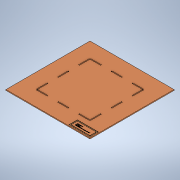
# Autodesk Inventor part: BasePlate_V1
Saved by Autodesk Inventor 2022.2 (Build 262287000, 287)
## iProperties
Created: 2022-11-15
Part Number: BasePlate_V1
Material: Generic
Document SubType Name: Modeling
Designer: jaege
Density: 1 g/cm^3
Appearance: Red Oak - Natural Low Gloss
Author: jaege
Autodesk Inventor part; units mm, degrees
(part 1 of 2)
ref_plane "YZ Plane" through (0, 0, 0) normal (1, 0, 0) x (0, 1, 0)
ref_plane "XZ Plane" through (0, 0, 0) normal (0, 1, 0) x (-1, 0, 0)
ref_plane "XY Plane" through (0, 0, 0) normal (0, 0, 1) x (1, 0, 0)
sketch "Sketch1" plane through (0, 0, 0) normal (0, 1, 0) x (-1, 0, 0)
  line L0 (200, -200) -> (-200, -200)
  line L1 (-200, -200) -> (-200, 200)
  line L2 (-200, 200) -> (200, 200)
  line L3 (200, 200) -> (200, -200)
  line L4 (200, -200) -> (-200, 200) construction
  line L5 (-200, -200) -> (200, 200) construction
  line L6 (-125, -125) -> (125, -125) construction
  line L7 (125, -125) -> (125, 125) construction
  line L8 (125, 125) -> (-125, 125) construction
  line L9 (-125, 125) -> (-125, -125) construction
  line L10 (-125, -125) -> (125, 125) construction
  line L11 (125, -125) -> (-125, 125) construction
  line L12 (125, 125) -> (129, 125)
  line L13 (129, 125) -> (129, 75)
  line L14 (129, 75) -> (125, 75)
  line L15 (125, 75) -> (125, 125)
  line L16 (125, 75) -> (129, 75)
  line L17 (125, 25) -> (125, 75) construction
  line L18 (129, 75) -> (129, 25) construction
  line L19 (129, 25) -> (125, 25)
  line L20 (125, 25) -> (129, 25)
  line L21 (125, -25) -> (125, 25)
  line L22 (129, 25) -> (129, -25)
  line L23 (129, -25) -> (125, -25)
  line L24 (125, -25) -> (129, -25)
  line L25 (125, -75) -> (125, -25) construction
  line L26 (129, -25) -> (129, -75) construction
  line L27 (129, -75) -> (125, -75)
  line L28 (125, -75) -> (129, -75)
  line L29 (125, -125) -> (125, -75)
  line L30 (129, -75) -> (129, -125)
  line L31 (129, -125) -> (125, -125)
  line L32 (125, 125) -> (75, 125)
  line L33 (75, 125) -> (75, 129)
  line L34 (75, 129) -> (125, 129)
  line L35 (125, 129) -> (125, 125)
  line L36 (125, -125) -> (75, -125)
  line L37 (75, -125) -> (75, -129)
  line L38 (75, -129) -> (125, -129)
  line L39 (125, -129) -> (125, -125)
  line L40 (75, 125) -> (25, 125) construction
  line L41 (75, 129) -> (75, 125)
  line L42 (25, 129) -> (75, 129) construction
  line L43 (25, 125) -> (25, 129)
  line L44 (75, -125) -> (25, -125) construction
  line L45 (25, -125) -> (25, -129)
  line L46 (25, -129) -> (75, -129) construction
  line L47 (75, -129) -> (75, -125)
  line L48 (25, 125) -> (-25, 125)
  line L49 (25, 129) -> (25, 125)
  line L50 (-25, 129) -> (25, 129)
  line L51 (-25, 125) -> (-25, 129)
  line L52 (25, -125) -> (-25, -125)
  line L53 (-25, -125) -> (-25, -129)
  line L54 (-25, -129) -> (25, -129)
  line L55 (25, -129) -> (25, -125)
  line L56 (-25, 125) -> (-75, 125) construction
  line L57 (-25, 129) -> (-25, 125)
  line L58 (-75, 129) -> (-25, 129) construction
  line L59 (-75, 125) -> (-75, 129)
  line L60 (-25, -125) -> (-75, -125) construction
  line L61 (-75, -125) -> (-75, -129)
  line L62 (-75, -129) -> (-25, -129) construction
  line L63 (-25, -129) -> (-25, -125)
  line L64 (-75, 125) -> (-125, 125)
  line L65 (-75, 129) -> (-75, 125)
  line L66 (-125, 129) -> (-75, 129)
  line L67 (-125, 125) -> (-125, 129)
  line L68 (-75, -125) -> (-125, -125)
  line L69 (-125, -125) -> (-125, -129)
  line L70 (-125, -129) -> (-75, -129)
  line L71 (-75, -129) -> (-75, -125)
  line L72 (-125, 125) -> (-129, 125)
  line L73 (-129, 125) -> (-129, 75)
  line L74 (-129, 75) -> (-125, 75)
  line L75 (-125, 75) -> (-125, 125)
  line L76 (-125, 25) -> (-125, 75)
  line L77 (-129, 25) -> (-125, 25)
  line L78 (-129, 75) -> (-129, 25) construction
  line L79 (-125, 75) -> (-129, 75)
  line L80 (-125, -25) -> (-125, 25)
  line L81 (-129, -25) -> (-125, -25)
  line L82 (-129, 25) -> (-129, -25)
  line L83 (-125, 25) -> (-129, 25)
  line L84 (-125, -75) -> (-125, -25) construction
  line L85 (-129, -75) -> (-125, -75)
  line L86 (-129, -25) -> (-129, -75) construction
  line L87 (-125, -25) -> (-129, -25)
  line L88 (-125, -125) -> (-125, -75)
  line L89 (-129, -125) -> (-125, -125)
  line L90 (-129, -75) -> (-129, -125)
  line L91 (-125, -75) -> (-129, -75)
  point P0 (0, 0)
  point P1 (75, -125)
  point P2 (25, -125)
  point P3 (-25, -125)
  point P4 (-75, -125)
  dimension "d0" = 400
  dimension "d1" = 400
  dimension "d2" = 250
  dimension "d3" = 250
  dimension "d4" = 4
  dimension "d5" = 50
  dimension "d8" = 50
  dimension "d13" = 50
  dimension "d14" = 4
  dimension "d15" = 50
  dimension "d16" = 4
  dimension "d19" = 50
  dimension "d24" = 4
  dimension "d25" = 50
  dimension "d28" = 50
  constraints: 184 end point, 12 parallel, 7 horizontal, 6 perpendicular, 4 midpoint, 2 vertical, 136 other
  measures "d0" distance of L1.end L2.end
  measures "d1" distance of L0.end L1.end
  measures "d2" distance of L8.end L7.end
  measures "d3" distance of L7.end L6.end
  measures "d4" distance of L13.end L14.end
  measures "d5" distance of L12.end L13.end
  measures "d8" distance of L12.end L16.end
  measures "d13" distance of L33.end L34.end
  measures "d14" distance of L32.end L33.end
  measures "d15" distance of L38.end L37.end
  measures "d16" distance of L37.end L36.end
  measures "d19" distance of L7.end L40.start
  measures "d24" distance of L74.end L73.end
  measures "d25" distance of L73.end L72.end
  measures "d28" distance of L74.end L76.start
extrude "Extrusion1" add sketch "Sketch1" along normal blind 4
sketch "Sketch2" plane through (0, 4, 0) normal (0, 1, 0) x (1, 0, 0)
  line L0 (-200, -200) -> (200, -200) projected
  line L1 (200, -200) -> (90, -200) construction
  line L2 (90, -200) -> (90, -150) construction
  line L3 (90, -150) -> (200, -150) construction
  line L4 (200, -150) -> (200, -200) construction
  line L5 (195, -155) -> (95, -155)
  line L6 (95, -155) -> (95, -195)
  line L7 (95, -195) -> (195, -195)
  line L8 (195, -195) -> (195, -155)
  line L9 (100, -160) -> (190, -160)
  line L10 (190, -160) -> (190, -190)
  line L11 (190, -190) -> (100, -190)
  line L12 (100, -190) -> (100, -160)
  line L13 (110, -168.25) -> (180, -168.25) construction
  line L14 (180, -168.25) -> (180, -181.75) construction
  line L15 (180, -181.75) -> (110, -181.75) construction
  line L16 (110, -181.75) -> (110, -168.25) construction
  line L17 (110, -168.25) -> (180, -181.75) construction
  line L18 (100, -190) -> (190, -160) construction
  spline S0 degree 2 poles (112.3777, -170.519) (112.3777, -170.7464) (112.2047, -171.0949) (112.0613, -171.2085) knots 0 0 0 1 2 2 2
  spline S1 degree 2 poles (112.0613, -171.2085) (111.8883, -171.342) (111.4953, -171.4557) (111.1839, -171.4557) knots 0 0 0 1 2 2 2
  line L19 (111.1839, -171.4557) -> (110.309, -171.4557)
  line L20 (110.309, -171.4557) -> (110.309, -168.4057)
  line L21 (110.309, -168.4057) -> (111.1172, -168.4057)
  spline S2 degree 2 poles (111.1172, -168.4057) (111.4434, -168.4057) (111.7697, -168.4477) (111.918, -168.5293) knots 0 0 0 1 2 2 2
  spline S3 degree 2 poles (111.918, -168.5293) (112.0836, -168.6158) (112.2344, -168.9) (112.2344, -169.0928) knots 0 0 0 1 2 2 2
  spline S4 degree 2 poles (112.2344, -169.0928) (112.2344, -169.3079) (112.007, -169.6489) (111.8068, -169.7453) knots 0 0 0 1 2 2 2
  line L22 (111.8068, -169.7453) -> (111.8068, -169.7602)
  spline S5 degree 2 poles (111.8068, -169.7602) (112.0786, -169.8343) (112.3777, -170.2273) (112.3777, -170.519) knots 0 0 0 1 2 2 2
  spline S6 degree 2 poles (111.9551, -170.5363) (111.9551, -170.3632) (111.8562, -170.1408) (111.7079, -170.0617) knots 0 0 0 1 2 2 2
  spline S7 degree 2 poles (111.7079, -170.0617) (111.6115, -170.0123) (111.3841, -169.9826) (111.174, -169.9826) knots 0 0 0 1 2 2 2
  line L23 (111.174, -169.9826) -> (110.7143, -169.9826)
  line L24 (110.7143, -169.9826) -> (110.7143, -171.1097)
  line L25 (110.7143, -171.1097) -> (111.043, -171.1097)
  spline S8 degree 2 poles (111.043, -171.1097) (111.31, -171.1097) (111.6165, -171.0603) (111.7351, -170.9812) knots 0 0 0 1 2 2 2
  spline S9 degree 2 poles (111.7351, -170.9812) (111.8488, -170.8996) (111.9551, -170.6969) (111.9551, -170.5363) knots 0 0 0 1 2 2 2
  spline S10 degree 2 poles (111.8117, -169.1497) (111.8117, -169.0409) (111.7376, -168.8778) (111.656, -168.8308) knots 0 0 0 1 2 2 2
  spline S11 degree 2 poles (111.656, -168.8308) (111.5571, -168.7765) (111.3174, -168.7517) (111.1024, -168.7517) knots 0 0 0 1 2 2 2
  line L26 (111.1024, -168.7517) -> (110.7143, -168.7517)
  line L27 (110.7143, -168.7517) -> (110.7143, -169.644)
  line L28 (110.7143, -169.644) -> (111.174, -169.644)
  spline S12 degree 2 poles (111.174, -169.644) (111.3643, -169.644) (111.5448, -169.6045) (111.6412, -169.5427) knots 0 0 0 1 2 2 2
  spline S13 degree 2 poles (111.6412, -169.5427) (111.7351, -169.4833) (111.8117, -169.293) (111.8117, -169.1497) knots 0 0 0 1 2 2 2
  spline S14 degree 2 poles (114.0263, -171.2135) (113.9793, -171.2481) (113.8212, -171.3717) (113.747, -171.4088) knots 0 0 0 1 2 2 2
  spline S15 degree 2 poles (113.747, -171.4088) (113.6457, -171.4631) (113.4553, -171.52) (113.2823, -171.52) knots 0 0 0 1 2 2 2
  spline S16 degree 2 poles (113.2823, -171.52) (113.1415, -171.52) (112.8869, -171.4137) (112.7905, -171.3173) knots 0 0 0 1 2 2 2
  spline S17 degree 2 poles (112.7905, -171.3173) (112.699, -171.2234) (112.5878, -170.9466) (112.5878, -170.7933) knots 0 0 0 1 2 2 2
  spline S18 degree 2 poles (112.5878, -170.7933) (112.5878, -170.556) (112.788, -170.2199) (113.0055, -170.1235) knots 0 0 0 1 2 2 2
  spline S19 degree 2 poles (113.0055, -170.1235) (113.1983, -170.0345) (113.7223, -169.9678) (114.0263, -169.9505) knots 0 0 0 1 2 2 2
  line L29 (114.0263, -169.9505) -> (114.0263, -169.8763)
  spline S20 degree 2 poles (114.0263, -169.8763) (114.0263, -169.7429) (113.9447, -169.5773) (113.8706, -169.5303) knots 0 0 0 1 2 2 2
  spline S21 degree 2 poles (113.8706, -169.5303) (113.7964, -169.4833) (113.5839, -169.4537) (113.4702, -169.4537) knots 0 0 0 1 2 2 2
  spline S22 degree 2 poles (113.4702, -169.4537) (113.3367, -169.4537) (112.9759, -169.5328) (112.7954, -169.6094) knots 0 0 0 1 2 2 2
  line L30 (112.7954, -169.6094) -> (112.7732, -169.6094)
  line L31 (112.7732, -169.6094) -> (112.7732, -169.2164)
  spline S23 degree 2 poles (112.7732, -169.2164) (112.8795, -169.1868) (113.2774, -169.1126) (113.4727, -169.1126) knots 0 0 0 1 2 2 2
  spline S24 degree 2 poles (113.4727, -169.1126) (113.7099, -169.1126) (114.0337, -169.1868) (114.1622, -169.2831) knots 0 0 0 1 2 2 2
  spline S25 degree 2 poles (114.1622, -169.2831) (114.2883, -169.3771) (114.4119, -169.6761) (114.4119, -169.8912) knots 0 0 0 1 2 2 2
  line L32 (114.4119, -169.8912) -> (114.4119, -171.4557)
  line L33 (114.4119, -171.4557) -> (114.0263, -171.4557)
  line L34 (114.0263, -171.4557) -> (114.0263, -171.2135)
  line L35 (114.0263, -170.8922) -> (114.0263, -170.257)
  spline S26 degree 2 poles (114.0263, -170.257) (113.8879, -170.2693) (113.4702, -170.3113) (113.3392, -170.3509) knots 0 0 0 1 2 2 2
  spline S27 degree 2 poles (113.3392, -170.3509) (113.1859, -170.3979) (112.9857, -170.5931) (112.9857, -170.7661) knots 0 0 0 1 2 2 2
  spline S28 degree 2 poles (112.9857, -170.7661) (112.9857, -170.9639) (113.2082, -171.1641) (113.4207, -171.1641) knots 0 0 0 1 2 2 2
  spline S29 degree 2 poles (113.4207, -171.1641) (113.6012, -171.1641) (113.8978, -171.0083) (114.0263, -170.8922) knots 0 0 0 1 2 2 2
  spline S30 degree 2 poles (115.8627, -171.5076) (115.6254, -171.5076) (115.2325, -171.3618) (115.0916, -171.2135) knots 0 0 0 1 2 2 2
  spline S31 degree 2 poles (115.0916, -171.2135) (114.9507, -171.0677) (114.795, -170.6178) (114.795, -170.3163) knots 0 0 0 1 2 2 2
  spline S32 degree 2 poles (114.795, -170.3163) (114.795, -170.0147) (114.9556, -169.5748) (115.0916, -169.4265) knots 0 0 0 1 2 2 2
  spline S33 degree 2 poles (115.0916, -169.4265) (115.2275, -169.2757) (115.6304, -169.1151) (115.8627, -169.1151) knots 0 0 0 1 2 2 2
  spline S34 degree 2 poles (115.8627, -169.1151) (116.0506, -169.1151) (116.4015, -169.2214) (116.5375, -169.2906) knots 0 0 0 1 2 2 2
  line L36 (116.5375, -169.2906) -> (116.5375, -169.7231)
  line L37 (116.5375, -169.7231) -> (116.5152, -169.7231)
  spline S35 degree 2 poles (116.5152, -169.7231) (116.4732, -169.6885) (116.3447, -169.5995) (116.2532, -169.5526) knots 0 0 0 1 2 2 2
  spline S36 degree 2 poles (116.2532, -169.5526) (116.1717, -169.513) (115.9542, -169.4512) (115.8553, -169.4512) knots 0 0 0 1 2 2 2
  spline S37 degree 2 poles (115.8553, -169.4512) (115.5562, -169.4512) (115.1929, -169.9035) (115.1929, -170.3163) knots 0 0 0 1 2 2 2
  spline S38 degree 2 poles (115.1929, -170.3163) (115.1929, -170.7192) (115.5439, -171.1715) (115.8553, -171.1715) knots 0 0 0 1 2 2 2
  spline S39 degree 2 poles (115.8553, -171.1715) (116.0432, -171.1715) (116.3842, -171.0158) (116.5152, -170.8947) knots 0 0 0 1 2 2 2
  line L38 (116.5152, -170.8947) -> (116.5375, -170.8947)
  line L39 (116.5375, -170.8947) -> (116.5375, -171.3272)
  spline S40 degree 2 poles (116.5375, -171.3272) (116.4806, -171.3544) (116.3076, -171.431) (116.2384, -171.4483) knots 0 0 0 1 2 2 2
  spline S41 degree 2 poles (116.2384, -171.4483) (116.1395, -171.478) (115.9838, -171.5076) (115.8627, -171.5076) knots 0 0 0 1 2 2 2
  line L40 (118.6853, -171.4557) -> (118.2998, -171.4557)
  line L41 (118.2998, -171.4557) -> (118.2998, -170.1507)
  spline S42 degree 2 poles (118.2998, -170.1507) (118.2998, -169.9925) (118.2701, -169.7206) (118.2256, -169.6391) knots 0 0 0 1 2 2 2
  spline S43 degree 2 poles (118.2256, -169.6391) (118.1786, -169.5526) (118.0106, -169.4685) (117.8672, -169.4685) knots 0 0 0 1 2 2 2
  spline S44 degree 2 poles (117.8672, -169.4685) (117.7239, -169.4685) (117.4199, -169.6218) (117.274, -169.7453) knots 0 0 0 1 2 2 2
  line L42 (117.274, -169.7453) -> (117.274, -171.4557)
  line L43 (117.274, -171.4557) -> (116.8885, -171.4557)
  line L44 (116.8885, -171.4557) -> (116.8885, -168.2698)
  line L45 (116.8885, -168.2698) -> (117.274, -168.2698)
  line L46 (117.274, -168.2698) -> (117.274, -169.4216)
  spline S45 degree 2 poles (117.274, -169.4216) (117.447, -169.2658) (117.7807, -169.1027) (117.9686, -169.1027) knots 0 0 0 1 2 2 2
  spline S46 degree 2 poles (117.9686, -169.1027) (118.3047, -169.1027) (118.6853, -169.5476) (118.6853, -169.9703) knots 0 0 0 1 2 2 2
  line L47 (118.6853, -169.9703) -> (118.6853, -171.4557)
  spline S47 degree 2 poles (120.2202, -171.5076) (119.6715, -171.5076) (119.0684, -170.8922) (119.0684, -170.3237) knots 0 0 0 1 2 2 2
  spline S48 degree 2 poles (119.0684, -170.3237) (119.0684, -169.7651) (119.6542, -169.1027) (120.1263, -169.1027) knots 0 0 0 1 2 2 2
  spline S49 degree 2 poles (120.1263, -169.1027) (120.3389, -169.1027) (120.6676, -169.2263) (120.7887, -169.3573) knots 0 0 0 1 2 2 2
  spline S50 degree 2 poles (120.7887, -169.3573) (120.9123, -169.4883) (121.0433, -169.8665) (121.0433, -170.1408) knots 0 0 0 1 2 2 2
  line L48 (121.0433, -170.1408) -> (121.0433, -170.3509)
  line L49 (121.0433, -170.3509) -> (119.459, -170.3509)
  spline S51 degree 2 poles (119.459, -170.3509) (119.459, -170.7488) (119.8594, -171.1715) (120.2153, -171.1715) knots 0 0 0 1 2 2 2
  spline S52 degree 2 poles (120.2153, -171.1715) (120.3413, -171.1715) (120.586, -171.1146) (120.6849, -171.0701) knots 0 0 0 1 2 2 2
  spline S53 degree 2 poles (120.6849, -171.0701) (120.7887, -171.0207) (120.9321, -170.9342) (120.979, -170.8947) knots 0 0 0 1 2 2 2
  line L50 (120.979, -170.8947) -> (121.0013, -170.8947)
  line L51 (121.0013, -170.8947) -> (121.0013, -171.3148)
  spline S54 degree 2 poles (121.0013, -171.3148) (120.9345, -171.342) (120.7318, -171.4211) (120.6528, -171.4434) knots 0 0 0 1 2 2 2
  spline S55 degree 2 poles (120.6528, -171.4434) (120.5415, -171.4755) (120.3586, -171.5076) (120.2202, -171.5076) knots 0 0 0 1 2 2 2
  spline S56 degree 2 poles (120.6676, -170.0568) (120.6626, -169.9011) (120.5984, -169.6737) (120.5366, -169.597) knots 0 0 0 1 2 2 2
  spline S57 degree 2 poles (120.5366, -169.597) (120.4699, -169.5105) (120.2598, -169.4191) (120.1041, -169.4191) knots 0 0 0 1 2 2 2
  spline S58 degree 2 poles (120.1041, -169.4191) (119.9508, -169.4191) (119.7358, -169.5105) (119.6468, -169.5995) knots 0 0 0 1 2 2 2
  spline S59 degree 2 poles (119.6468, -169.5995) (119.5603, -169.691) (119.4713, -169.9109) (119.459, -170.0568) knots 0 0 0 1 2 2 2
  line L52 (119.459, -170.0568) -> (120.6676, -170.0568)
  line L53 (121.8268, -171.4557) -> (121.4412, -171.4557)
  line L54 (121.4412, -171.4557) -> (121.4412, -168.2698)
  line L55 (121.4412, -168.2698) -> (121.8268, -168.2698)
  line L56 (121.8268, -168.2698) -> (121.8268, -171.4557)
  spline S60 degree 2 poles (124.2737, -170.3113) (124.2737, -170.8897) (123.7176, -171.52) (123.2529, -171.52) knots 0 0 0 1 2 2 2
  spline S61 degree 2 poles (123.2529, -171.52) (122.7759, -171.52) (122.2297, -170.8699) (122.2297, -170.3113) knots 0 0 0 1 2 2 2
  spline S62 degree 2 poles (122.2297, -170.3113) (122.2297, -169.7379) (122.7932, -169.1027) (123.2529, -169.1027) knots 0 0 0 1 2 2 2
  spline S63 degree 2 poles (123.2529, -169.1027) (123.7176, -169.1027) (124.2737, -169.7355) (124.2737, -170.3113) knots 0 0 0 1 2 2 2
  spline S64 degree 2 poles (123.8758, -170.3113) (123.8758, -169.8665) (123.552, -169.4339) (123.2529, -169.4339) knots 0 0 0 1 2 2 2
  spline S65 degree 2 poles (123.2529, -169.4339) (122.9538, -169.4339) (122.6276, -169.8665) (122.6276, -170.3113) knots 0 0 0 1 2 2 2
  spline S66 degree 2 poles (122.6276, -170.3113) (122.6276, -170.7439) (122.9538, -171.1888) (123.2529, -171.1888) knots 0 0 0 1 2 2 2
  spline S67 degree 2 poles (123.2529, -171.1888) (123.5495, -171.1888) (123.8758, -170.7513) (123.8758, -170.3113) knots 0 0 0 1 2 2 2
  line L57 (125.8827, -169.5797) -> (125.863, -169.5797)
  spline S68 degree 2 poles (125.863, -169.5797) (125.8185, -169.5674) (125.7221, -169.5624) (125.6553, -169.5624) knots 0 0 0 1 2 2 2
  spline S69 degree 2 poles (125.6553, -169.5624) (125.4996, -169.5624) (125.1932, -169.6984) (125.0547, -169.8318) knots 0 0 0 1 2 2 2
  line L58 (125.0547, -169.8318) -> (125.0547, -171.4557)
  line L59 (125.0547, -171.4557) -> (124.6692, -171.4557)
  line L60 (124.6692, -171.4557) -> (124.6692, -169.167)
  line L61 (124.6692, -169.167) -> (125.0547, -169.167)
  line L62 (125.0547, -169.167) -> (125.0547, -169.5081)
  spline S70 degree 2 poles (125.0547, -169.5081) (125.2648, -169.3202) (125.5787, -169.167) (125.727, -169.167) knots 0 0 0 1 2 2 2
  spline S71 degree 2 poles (125.727, -169.167) (125.7863, -169.167) (125.8457, -169.1719) (125.8827, -169.1793) knots 0 0 0 1 2 2 2
  line L63 (125.8827, -169.1793) -> (125.8827, -169.5797)
  spline S72 degree 2 poles (128.0998, -170.2496) (128.0998, -170.823) (127.5536, -171.5002) (127.1359, -171.5002) knots 0 0 0 1 2 2 2
  spline S73 degree 2 poles (127.1359, -171.5002) (126.9653, -171.5002) (126.7033, -171.4211) (126.5674, -171.3395) knots 0 0 0 1 2 2 2
  line L64 (126.5674, -171.3395) -> (126.5674, -172.2985)
  line L65 (126.5674, -172.2985) -> (126.1818, -172.2985)
  line L66 (126.1818, -172.2985) -> (126.1818, -169.167)
  line L67 (126.1818, -169.167) -> (126.5674, -169.167)
  line L68 (126.5674, -169.167) -> (126.5674, -169.4067)
  spline S74 degree 2 poles (126.5674, -169.4067) (126.7107, -169.2757) (127.0617, -169.1027) (127.2669, -169.1027) knots 0 0 0 1 2 2 2
  spline S75 degree 2 poles (127.2669, -169.1027) (127.6598, -169.1027) (128.0998, -169.7256) (128.0998, -170.2496) knots 0 0 0 1 2 2 2
  spline S76 degree 2 poles (127.7019, -170.294) (127.7019, -169.9011) (127.4522, -169.4685) (127.1729, -169.4685) knots 0 0 0 1 2 2 2
  spline S77 degree 2 poles (127.1729, -169.4685) (127.0098, -169.4685) (126.7033, -169.6143) (126.5674, -169.728) knots 0 0 0 1 2 2 2
  line L69 (126.5674, -169.728) -> (126.5674, -171.0281)
  spline S78 degree 2 poles (126.5674, -171.0281) (126.7182, -171.0998) (126.9332, -171.1542) (127.0716, -171.1542) knots 0 0 0 1 2 2 2
  spline S79 degree 2 poles (127.0716, -171.1542) (127.3707, -171.1542) (127.7019, -170.7142) (127.7019, -170.294) knots 0 0 0 1 2 2 2
  line L70 (129.7138, -169.5797) -> (129.694, -169.5797)
  spline S80 degree 2 poles (129.694, -169.5797) (129.6495, -169.5674) (129.5531, -169.5624) (129.4864, -169.5624) knots 0 0 0 1 2 2 2
  spline S81 degree 2 poles (129.4864, -169.5624) (129.3307, -169.5624) (129.0242, -169.6984) (128.8858, -169.8318) knots 0 0 0 1 2 2 2
  line L71 (128.8858, -169.8318) -> (128.8858, -171.4557)
  line L72 (128.8858, -171.4557) -> (128.5002, -171.4557)
  line L73 (128.5002, -171.4557) -> (128.5002, -169.167)
  line L74 (128.5002, -169.167) -> (128.8858, -169.167)
  line L75 (128.8858, -169.167) -> (128.8858, -169.5081)
  spline S82 degree 2 poles (128.8858, -169.5081) (129.0959, -169.3202) (129.4098, -169.167) (129.5581, -169.167) knots 0 0 0 1 2 2 2
  spline S83 degree 2 poles (129.5581, -169.167) (129.6174, -169.167) (129.6767, -169.1719) (129.7138, -169.1793) knots 0 0 0 1 2 2 2
  line L76 (129.7138, -169.1793) -> (129.7138, -169.5797)
  spline S84 degree 2 poles (131.8938, -170.3113) (131.8938, -170.8897) (131.3376, -171.52) (130.873, -171.52) knots 0 0 0 1 2 2 2
  spline S85 degree 2 poles (130.873, -171.52) (130.3959, -171.52) (129.8497, -170.8699) (129.8497, -170.3113) knots 0 0 0 1 2 2 2
  spline S86 degree 2 poles (129.8497, -170.3113) (129.8497, -169.7379) (130.4133, -169.1027) (130.873, -169.1027) knots 0 0 0 1 2 2 2
  spline S87 degree 2 poles (130.873, -169.1027) (131.3376, -169.1027) (131.8938, -169.7355) (131.8938, -170.3113) knots 0 0 0 1 2 2 2
  spline S88 degree 2 poles (131.4958, -170.3113) (131.4958, -169.8665) (131.172, -169.4339) (130.873, -169.4339) knots 0 0 0 1 2 2 2
  spline S89 degree 2 poles (130.873, -169.4339) (130.5739, -169.4339) (130.2477, -169.8665) (130.2477, -170.3113) knots 0 0 0 1 2 2 2
  spline S90 degree 2 poles (130.2477, -170.3113) (130.2477, -170.7439) (130.5739, -171.1888) (130.873, -171.1888) knots 0 0 0 1 2 2 2
  spline S91 degree 2 poles (130.873, -171.1888) (131.1696, -171.1888) (131.4958, -170.7513) (131.4958, -170.3113) knots 0 0 0 1 2 2 2
  spline S92 degree 2 poles (133.2828, -171.5076) (132.7341, -171.5076) (132.131, -170.8922) (132.131, -170.3237) knots 0 0 0 1 2 2 2
  spline S93 degree 2 poles (132.131, -170.3237) (132.131, -169.7651) (132.7168, -169.1027) (133.1889, -169.1027) knots 0 0 0 1 2 2 2
  spline S94 degree 2 poles (133.1889, -169.1027) (133.4015, -169.1027) (133.7302, -169.2263) (133.8513, -169.3573) knots 0 0 0 1 2 2 2
  spline S95 degree 2 poles (133.8513, -169.3573) (133.9749, -169.4883) (134.1059, -169.8665) (134.1059, -170.1408) knots 0 0 0 1 2 2 2
  line L77 (134.1059, -170.1408) -> (134.1059, -170.3509)
  line L78 (134.1059, -170.3509) -> (132.5216, -170.3509)
  spline S96 degree 2 poles (132.5216, -170.3509) (132.5216, -170.7488) (132.922, -171.1715) (133.2779, -171.1715) knots 0 0 0 1 2 2 2
  spline S97 degree 2 poles (133.2779, -171.1715) (133.4039, -171.1715) (133.6486, -171.1146) (133.7475, -171.0701) knots 0 0 0 1 2 2 2
  spline S98 degree 2 poles (133.7475, -171.0701) (133.8513, -171.0207) (133.9947, -170.9342) (134.0416, -170.8947) knots 0 0 0 1 2 2 2
  line L79 (134.0416, -170.8947) -> (134.0639, -170.8947)
  line L80 (134.0639, -170.8947) -> (134.0639, -171.3148)
  spline S99 degree 2 poles (134.0639, -171.3148) (133.9971, -171.342) (133.7944, -171.4211) (133.7154, -171.4434) knots 0 0 0 1 2 2 2
  spline S100 degree 2 poles (133.7154, -171.4434) (133.6041, -171.4755) (133.4212, -171.5076) (133.2828, -171.5076) knots 0 0 0 1 2 2 2
  spline S101 degree 2 poles (133.7302, -170.0568) (133.7252, -169.9011) (133.661, -169.6737) (133.5992, -169.597) knots 0 0 0 1 2 2 2
  spline S102 degree 2 poles (133.5992, -169.597) (133.5325, -169.5105) (133.3224, -169.4191) (133.1667, -169.4191) knots 0 0 0 1 2 2 2
  spline S103 degree 2 poles (133.1667, -169.4191) (133.0134, -169.4191) (132.7984, -169.5105) (132.7094, -169.5995) knots 0 0 0 1 2 2 2
  spline S104 degree 2 poles (132.7094, -169.5995) (132.6229, -169.691) (132.5339, -169.9109) (132.5216, -170.0568) knots 0 0 0 1 2 2 2
  line L81 (132.5216, -170.0568) -> (133.7302, -170.0568)
  line L82 (135.7001, -168.6405) -> (135.6803, -168.6405)
  spline S105 degree 2 poles (135.6803, -168.6405) (135.6284, -168.6207) (135.4356, -168.5861) (135.359, -168.5861) knots 0 0 0 1 2 2 2
  spline S106 degree 2 poles (135.359, -168.5861) (135.1168, -168.5861) (134.9092, -168.8036) (134.9092, -169.0904) knots 0 0 0 1 2 2 2
  line L83 (134.9092, -169.0904) -> (134.9092, -169.167)
  line L84 (134.9092, -169.167) -> (135.5468, -169.167)
  line L85 (135.5468, -169.167) -> (135.5468, -169.4858)
  line L86 (135.5468, -169.4858) -> (134.9215, -169.4858)
  line L87 (134.9215, -169.4858) -> (134.9215, -171.4557)
  line L88 (134.9215, -171.4557) -> (134.5359, -171.4557)
  line L89 (134.5359, -171.4557) -> (134.5359, -169.4858)
  line L90 (134.5359, -169.4858) -> (134.2764, -169.4858)
  line L91 (134.2764, -169.4858) -> (134.2764, -169.167)
  line L92 (134.2764, -169.167) -> (134.5359, -169.167)
  line L93 (134.5359, -169.167) -> (134.5359, -169.0904)
  spline S107 degree 2 poles (134.5359, -169.0904) (134.5359, -168.6801) (134.9339, -168.25) (135.3046, -168.25) knots 0 0 0 1 2 2 2
  spline S108 degree 2 poles (135.3046, -168.25) (135.4109, -168.25) (135.616, -168.2722) (135.7001, -168.2871) knots 0 0 0 1 2 2 2
  line L94 (135.7001, -168.2871) -> (135.7001, -168.6405)
  line L95 (111.0201, -176.4749) -> (111.0201, -173.7876)
  line L96 (111.0201, -173.7876) -> (109.9975, -173.7876)
  line L97 (109.9975, -173.7876) -> (109.9975, -173.4269)
  line L98 (109.9975, -173.4269) -> (112.4478, -173.4269)
  line L99 (112.4478, -173.4269) -> (112.4478, -173.7876)
  line L100 (112.4478, -173.7876) -> (111.4252, -173.7876)
  line L101 (111.4252, -173.7876) -> (111.4252, -176.4749)
  line L102 (111.4252, -176.4749) -> (111.0201, -176.4749)
  line L103 (113.1196, -176.4749) -> (112.7343, -176.4749)
  line L104 (112.7343, -176.4749) -> (112.7343, -174.1877)
  line L105 (112.7343, -174.1877) -> (113.1196, -174.1877)
  line L106 (113.1196, -174.1877) -> (113.1196, -176.4749)
  line L107 (113.1468, -173.8073) -> (112.7096, -173.8073)
  line L108 (112.7096, -173.8073) -> (112.7096, -173.4072)
  line L109 (112.7096, -173.4072) -> (113.1468, -173.4072)
  line L110 (113.1468, -173.4072) -> (113.1468, -173.8073)
  line L111 (116.2788, -176.4749) -> (116.2788, -175.151)
  spline S109 degree 2 poles (116.2788, -175.151) (116.2788, -174.9929) (116.2541, -174.7237) (116.2146, -174.6496) knots 0 0 0 1 2 2 2
  spline S110 degree 2 poles (116.2146, -174.6496) (116.175, -174.5681) (116.0244, -174.489) (115.8935, -174.489) knots 0 0 0 1 2 2 2
  spline S111 degree 2 poles (115.8935, -174.489) (115.7749, -174.489) (115.5032, -174.6348) (115.3599, -174.7731) knots 0 0 0 1 2 2 2
  spline S112 degree 2 poles (115.3599, -174.7731) (115.3624, -174.8077) (115.3673, -174.904) (115.3673, -174.9682) knots 0 0 0 1 2 2 2
  line L112 (115.3673, -174.9682) -> (115.3673, -176.4749)
  line L113 (115.3673, -176.4749) -> (114.982, -176.4749)
  line L114 (114.982, -176.4749) -> (114.982, -175.151)
  spline S113 degree 2 poles (114.982, -175.151) (114.982, -174.9929) (114.9573, -174.7237) (114.9178, -174.6496) knots 0 0 0 1 2 2 2
  spline S114 degree 2 poles (114.9178, -174.6496) (114.8783, -174.5681) (114.7276, -174.489) (114.5967, -174.489) knots 0 0 0 1 2 2 2
  spline S115 degree 2 poles (114.5967, -174.489) (114.4732, -174.489) (114.199, -174.6447) (114.0706, -174.7657) knots 0 0 0 1 2 2 2
  line L115 (114.0706, -174.7657) -> (114.0706, -176.4749)
  line L116 (114.0706, -176.4749) -> (113.6853, -176.4749)
  line L117 (113.6853, -176.4749) -> (113.6853, -174.1877)
  line L118 (113.6853, -174.1877) -> (114.0706, -174.1877)
  line L119 (114.0706, -174.1877) -> (114.0706, -174.4396)
  spline S116 degree 2 poles (114.0706, -174.4396) (114.2213, -174.289) (114.5177, -174.1235) (114.6955, -174.1235) knots 0 0 0 1 2 2 2
  spline S117 degree 2 poles (114.6955, -174.1235) (114.898, -174.1235) (115.2117, -174.3087) (115.2932, -174.5187) knots 0 0 0 1 2 2 2
  spline S118 degree 2 poles (115.2932, -174.5187) (115.4686, -174.3236) (115.7996, -174.1235) (115.9923, -174.1235) knots 0 0 0 1 2 2 2
  spline S119 degree 2 poles (115.9923, -174.1235) (116.1405, -174.1235) (116.3825, -174.2149) (116.4714, -174.3186) knots 0 0 0 1 2 2 2
  spline S120 degree 2 poles (116.4714, -174.3186) (116.5628, -174.4224) (116.6641, -174.7336) (116.6641, -174.9682) knots 0 0 0 1 2 2 2
  line L120 (116.6641, -174.9682) -> (116.6641, -176.4749)
  line L121 (116.6641, -176.4749) -> (116.2788, -176.4749)
  spline S121 degree 2 poles (119.6923, -175.6821) (119.6923, -176.0822) (119.2033, -176.5169) (118.7908, -176.5169) knots 0 0 0 1 2 2 2
  spline S122 degree 2 poles (118.7908, -176.5169) (118.692, -176.5169) (118.3635, -176.4823) (118.2523, -176.4576) knots 0 0 0 1 2 2 2
  line L122 (118.2523, -176.4576) -> (118.2523, -176.0674)
  line L123 (118.2523, -176.0674) -> (118.2746, -176.0674)
  spline S123 degree 2 poles (118.2746, -176.0674) (118.3585, -176.097) (118.608, -176.1662) (118.7364, -176.1662) knots 0 0 0 1 2 2 2
  spline S124 degree 2 poles (118.7364, -176.1662) (118.9242, -176.1662) (119.1489, -176.0797) (119.2008, -176.0007) knots 0 0 0 1 2 2 2
  spline S125 degree 2 poles (119.2008, -176.0007) (119.2576, -175.9192) (119.2873, -175.6821) (119.2873, -175.5265) knots 0 0 0 1 2 2 2
  line L124 (119.2873, -175.5265) -> (119.2873, -173.7505)
  line L125 (119.2873, -173.7505) -> (118.6426, -173.7505)
  line L126 (118.6426, -173.7505) -> (118.6426, -173.4269)
  line L127 (118.6426, -173.4269) -> (119.6923, -173.4269)
  line L128 (119.6923, -173.4269) -> (119.6923, -175.6821)
  spline S126 degree 2 poles (121.535, -176.2329) (121.488, -176.2675) (121.33, -176.391) (121.2559, -176.428) knots 0 0 0 1 2 2 2
  spline S127 degree 2 poles (121.2559, -176.428) (121.1546, -176.4823) (120.9644, -176.5392) (120.7915, -176.5392) knots 0 0 0 1 2 2 2
  spline S128 degree 2 poles (120.7915, -176.5392) (120.6507, -176.5392) (120.3963, -176.4329) (120.3, -176.3366) knots 0 0 0 1 2 2 2
  spline S129 degree 2 poles (120.3, -176.3366) (120.2086, -176.2428) (120.0974, -175.9661) (120.0974, -175.813) knots 0 0 0 1 2 2 2
  spline S130 degree 2 poles (120.0974, -175.813) (120.0974, -175.5759) (120.2975, -175.2399) (120.5149, -175.1436) knots 0 0 0 1 2 2 2
  spline S131 degree 2 poles (120.5149, -175.1436) (120.7075, -175.0547) (121.2312, -174.988) (121.535, -174.9707) knots 0 0 0 1 2 2 2
  line L129 (121.535, -174.9707) -> (121.535, -174.8966)
  spline S132 degree 2 poles (121.535, -174.8966) (121.535, -174.7632) (121.4535, -174.5977) (121.3794, -174.5508) knots 0 0 0 1 2 2 2
  spline S133 degree 2 poles (121.3794, -174.5508) (121.3053, -174.5039) (121.0928, -174.4742) (120.9792, -174.4742) knots 0 0 0 1 2 2 2
  spline S134 degree 2 poles (120.9792, -174.4742) (120.8458, -174.4742) (120.4852, -174.5533) (120.3049, -174.6298) knots 0 0 0 1 2 2 2
  line L130 (120.3049, -174.6298) -> (120.2827, -174.6298)
  line L131 (120.2827, -174.6298) -> (120.2827, -174.2371)
  spline S135 degree 2 poles (120.2827, -174.2371) (120.3889, -174.2075) (120.7866, -174.1334) (120.9817, -174.1334) knots 0 0 0 1 2 2 2
  spline S136 degree 2 poles (120.9817, -174.1334) (121.2188, -174.1334) (121.5424, -174.2075) (121.6708, -174.3038) knots 0 0 0 1 2 2 2
  spline S137 degree 2 poles (121.6708, -174.3038) (121.7968, -174.3977) (121.9203, -174.6965) (121.9203, -174.9114) knots 0 0 0 1 2 2 2
  line L132 (121.9203, -174.9114) -> (121.9203, -176.4749)
  line L133 (121.9203, -176.4749) -> (121.535, -176.4749)
  line L134 (121.535, -176.4749) -> (121.535, -176.2329)
  line L135 (121.535, -175.9118) -> (121.535, -175.277)
  spline S138 degree 2 poles (121.535, -175.277) (121.3967, -175.2893) (120.9792, -175.3313) (120.8483, -175.3708) knots 0 0 0 1 2 2 2
  spline S139 degree 2 poles (120.8483, -175.3708) (120.6952, -175.4178) (120.4951, -175.6129) (120.4951, -175.7858) knots 0 0 0 1 2 2 2
  spline S140 degree 2 poles (120.4951, -175.7858) (120.4951, -175.9834) (120.7174, -176.1835) (120.9298, -176.1835) knots 0 0 0 1 2 2 2
  spline S141 degree 2 poles (120.9298, -176.1835) (121.1101, -176.1835) (121.4065, -176.0279) (121.535, -175.9118) knots 0 0 0 1 2 2 2
  line L136 (121.6881, -173.8048) -> (121.2756, -173.8048)
  line L137 (121.2756, -173.8048) -> (121.2756, -173.4047)
  line L138 (121.2756, -173.4047) -> (121.6881, -173.4047)
  line L139 (121.6881, -173.4047) -> (121.6881, -173.8048)
  line L140 (120.8434, -173.8048) -> (120.4309, -173.8048)
  line L141 (120.4309, -173.8048) -> (120.4309, -173.4047)
  line L142 (120.4309, -173.4047) -> (120.8434, -173.4047)
  line L143 (120.8434, -173.4047) -> (120.8434, -173.8048)
  spline S142 degree 2 poles (122.5427, -176.8405) (122.5823, -176.8578) (122.7329, -176.9121) (122.8293, -176.9344) knots 0 0 0 1 2 2 2
  spline S143 degree 2 poles (122.8293, -176.9344) (122.9355, -176.9615) (123.1158, -176.9936) (123.222, -176.9936) knots 0 0 0 1 2 2 2
  spline S144 degree 2 poles (123.222, -176.9936) (123.3998, -176.9936) (123.6468, -176.8998) (123.716, -176.8158) knots 0 0 0 1 2 2 2
  spline S145 degree 2 poles (123.716, -176.8158) (123.7827, -176.7318) (123.8346, -176.512) (123.8346, -176.3712) knots 0 0 0 1 2 2 2
  line L144 (123.8346, -176.3712) -> (123.8346, -176.1711)
  spline S146 degree 2 poles (123.8346, -176.1711) (123.6789, -176.307) (123.3801, -176.4354) (123.1553, -176.4354) knots 0 0 0 1 2 2 2
  spline S147 degree 2 poles (123.1553, -176.4354) (122.765, -176.4354) (122.3032, -175.855) (122.3032, -175.3091) knots 0 0 0 1 2 2 2
  spline S148 degree 2 poles (122.3032, -175.3091) (122.3032, -175.025) (122.4637, -174.5854) (122.5971, -174.4298) knots 0 0 0 1 2 2 2
  spline S149 degree 2 poles (122.5971, -174.4298) (122.7255, -174.284) (123.0787, -174.1235) (123.2665, -174.1235) knots 0 0 0 1 2 2 2
  spline S150 degree 2 poles (123.2665, -174.1235) (123.4443, -174.1235) (123.7037, -174.2075) (123.8346, -174.284) knots 0 0 0 1 2 2 2
  line L145 (123.8346, -174.284) -> (123.8568, -174.1877)
  line L146 (123.8568, -174.1877) -> (124.2199, -174.1877)
  line L147 (124.2199, -174.1877) -> (124.2199, -176.2131)
  spline S151 degree 2 poles (124.2199, -176.2131) (124.2199, -176.796) (123.7135, -177.3394) (123.1924, -177.3394) knots 0 0 0 1 2 2 2
  spline S152 degree 2 poles (123.1924, -177.3394) (123.0244, -177.3394) (122.6737, -177.2851) (122.523, -177.2406) knots 0 0 0 1 2 2 2
  line L148 (122.523, -177.2406) -> (122.523, -176.8405)
  line L149 (122.523, -176.8405) -> (122.5427, -176.8405)
  line L150 (123.8346, -175.855) -> (123.8346, -174.5977)
  spline S153 degree 2 poles (123.8346, -174.5977) (123.6913, -174.5286) (123.4492, -174.4693) (123.3282, -174.4693) knots 0 0 0 1 2 2 2
  spline S154 degree 2 poles (123.3282, -174.4693) (123.0367, -174.4693) (122.7008, -174.8991) (122.7008, -175.3017) knots 0 0 0 1 2 2 2
  spline S155 degree 2 poles (122.7008, -175.3017) (122.7008, -175.6821) (122.9552, -176.0797) (123.2418, -176.0797) knots 0 0 0 1 2 2 2
  spline S156 degree 2 poles (123.2418, -176.0797) (123.3924, -176.0797) (123.7086, -175.9612) (123.8346, -175.855) knots 0 0 0 1 2 2 2
  spline S157 degree 2 poles (125.7711, -176.5268) (125.2227, -176.5268) (124.62, -175.9118) (124.62, -175.3437) knots 0 0 0 1 2 2 2
  spline S158 degree 2 poles (124.62, -175.3437) (124.62, -174.7854) (125.2054, -174.1235) (125.6772, -174.1235) knots 0 0 0 1 2 2 2
  spline S159 degree 2 poles (125.6772, -174.1235) (125.8896, -174.1235) (126.2181, -174.247) (126.3392, -174.3779) knots 0 0 0 1 2 2 2
  spline S160 degree 2 poles (126.3392, -174.3779) (126.4627, -174.5088) (126.5936, -174.8867) (126.5936, -175.1609) knots 0 0 0 1 2 2 2
  line L151 (126.5936, -175.1609) -> (126.5936, -175.3708)
  line L152 (126.5936, -175.3708) -> (125.0103, -175.3708)
  spline S161 degree 2 poles (125.0103, -175.3708) (125.0103, -175.7685) (125.4104, -176.1909) (125.7661, -176.1909) knots 0 0 0 1 2 2 2
  spline S162 degree 2 poles (125.7661, -176.1909) (125.8921, -176.1909) (126.1366, -176.1341) (126.2354, -176.0896) knots 0 0 0 1 2 2 2
  spline S163 degree 2 poles (126.2354, -176.0896) (126.3392, -176.0402) (126.4824, -175.9538) (126.5293, -175.9142) knots 0 0 0 1 2 2 2
  line L153 (126.5293, -175.9142) -> (126.5516, -175.9142)
  line L154 (126.5516, -175.9142) -> (126.5516, -176.3341)
  spline S164 degree 2 poles (126.5516, -176.3341) (126.4849, -176.3613) (126.2823, -176.4404) (126.2033, -176.4626) knots 0 0 0 1 2 2 2
  spline S165 degree 2 poles (126.2033, -176.4626) (126.0922, -176.4947) (125.9094, -176.5268) (125.7711, -176.5268) knots 0 0 0 1 2 2 2
  spline S166 degree 2 poles (126.2181, -175.0769) (126.2132, -174.9213) (126.149, -174.6941) (126.0872, -174.6175) knots 0 0 0 1 2 2 2
  spline S167 degree 2 poles (126.0872, -174.6175) (126.0205, -174.531) (125.8106, -174.4396) (125.655, -174.4396) knots 0 0 0 1 2 2 2
  spline S168 degree 2 poles (125.655, -174.4396) (125.5018, -174.4396) (125.2869, -174.531) (125.198, -174.62) knots 0 0 0 1 2 2 2
  spline S169 degree 2 poles (125.198, -174.62) (125.1116, -174.7113) (125.0226, -174.9312) (125.0103, -175.0769) knots 0 0 0 1 2 2 2
  line L155 (125.0103, -175.0769) -> (126.2181, -175.0769)
  line L156 (128.1966, -174.6002) -> (128.1768, -174.6002)
  spline S170 degree 2 poles (128.1768, -174.6002) (128.1324, -174.5878) (128.0361, -174.5829) (127.9694, -174.5829) knots 0 0 0 1 2 2 2
  spline S171 degree 2 poles (127.9694, -174.5829) (127.8138, -174.5829) (127.5075, -174.7188) (127.3692, -174.8521) knots 0 0 0 1 2 2 2
  line L157 (127.3692, -174.8521) -> (127.3692, -176.4749)
  line L158 (127.3692, -176.4749) -> (126.9838, -176.4749)
  line L159 (126.9838, -176.4749) -> (126.9838, -174.1877)
  line L160 (126.9838, -174.1877) -> (127.3692, -174.1877)
  line L161 (127.3692, -174.1877) -> (127.3692, -174.5286)
  spline S172 degree 2 poles (127.3692, -174.5286) (127.5791, -174.3408) (127.8928, -174.1877) (128.041, -174.1877) knots 0 0 0 1 2 2 2
  spline S173 degree 2 poles (128.041, -174.1877) (128.1003, -174.1877) (128.1596, -174.1926) (128.1966, -174.2001) knots 0 0 0 1 2 2 2
  line L162 (128.1966, -174.2001) -> (128.1966, -174.6002)
  line L163 (111.3709, -181.4934) -> (110.1902, -181.4934)
  line L164 (110.1902, -181.4934) -> (110.1902, -181.1822)
  line L165 (110.1902, -181.1822) -> (110.578, -181.1822)
  line L166 (110.578, -181.1822) -> (110.578, -178.7566)
  line L167 (110.578, -178.7566) -> (110.1902, -178.7566)
  line L168 (110.1902, -178.7566) -> (110.1902, -178.4454)
  line L169 (110.1902, -178.4454) -> (111.3709, -178.4454)
  line L170 (111.3709, -178.4454) -> (111.3709, -178.7566)
  line L171 (111.3709, -178.7566) -> (110.9831, -178.7566)
  line L172 (110.9831, -178.7566) -> (110.9831, -181.1822)
  line L173 (110.9831, -181.1822) -> (111.3709, -181.1822)
  line L174 (111.3709, -181.1822) -> (111.3709, -181.4934)
  line L175 (113.6383, -181.4934) -> (113.253, -181.4934)
  line L176 (113.253, -181.4934) -> (113.253, -180.1892)
  spline S174 degree 2 poles (113.253, -180.1892) (113.253, -180.0311) (113.2234, -179.7594) (113.1789, -179.6779) knots 0 0 0 1 2 2 2
  spline S175 degree 2 poles (113.1789, -179.6779) (113.132, -179.5915) (112.964, -179.5075) (112.8208, -179.5075) knots 0 0 0 1 2 2 2
  spline S176 degree 2 poles (112.8208, -179.5075) (112.6775, -179.5075) (112.3737, -179.6606) (112.228, -179.7841) knots 0 0 0 1 2 2 2
  line L177 (112.228, -179.7841) -> (112.228, -181.4934)
  line L178 (112.228, -181.4934) -> (111.8426, -181.4934)
  line L179 (111.8426, -181.4934) -> (111.8426, -179.2062)
  line L180 (111.8426, -179.2062) -> (112.228, -179.2062)
  line L181 (112.228, -179.2062) -> (112.228, -179.4606)
  spline S177 degree 2 poles (112.228, -179.4606) (112.4009, -179.305) (112.7343, -179.1419) (112.922, -179.1419) knots 0 0 0 1 2 2 2
  spline S178 degree 2 poles (112.922, -179.1419) (113.258, -179.1419) (113.6383, -179.5865) (113.6383, -180.0089) knots 0 0 0 1 2 2 2
  line L182 (113.6383, -180.0089) -> (113.6383, -181.4934)
  line L183 (115.9379, -181.4934) -> (115.5526, -181.4934)
  line L184 (115.5526, -181.4934) -> (115.5526, -181.2612)
  spline S179 degree 2 poles (115.5526, -181.2612) (115.4637, -181.3353) (115.3328, -181.4341) (115.2438, -181.4761) knots 0 0 0 1 2 2 2
  spline S180 degree 2 poles (115.2438, -181.4761) (115.1623, -181.5156) (114.987, -181.5576) (114.8709, -181.5576) knots 0 0 0 1 2 2 2
  spline S181 degree 2 poles (114.8709, -181.5576) (114.6832, -181.5576) (114.367, -181.402) (114.2558, -181.2513) knots 0 0 0 1 2 2 2
  spline S182 degree 2 poles (114.2558, -181.2513) (114.1447, -181.1007) (114.0212, -180.6561) (114.0212, -180.3671) knots 0 0 0 1 2 2 2
  spline S183 degree 2 poles (114.0212, -180.3671) (114.0212, -180.0657) (114.1768, -179.6261) (114.3126, -179.4606) knots 0 0 0 1 2 2 2
  spline S184 degree 2 poles (114.3126, -179.4606) (114.4386, -179.3124) (114.7918, -179.1419) (114.987, -179.1419) knots 0 0 0 1 2 2 2
  spline S185 degree 2 poles (114.987, -179.1419) (115.1574, -179.1419) (115.4118, -179.2185) (115.5526, -179.2975) knots 0 0 0 1 2 2 2
  line L185 (115.5526, -179.2975) -> (115.5526, -178.3095)
  line L186 (115.5526, -178.3095) -> (115.9379, -178.3095)
  line L187 (115.9379, -178.3095) -> (115.9379, -181.4934)
  line L188 (115.5526, -180.9376) -> (115.5526, -179.6162)
  spline S186 degree 2 poles (115.5526, -179.6162) (115.4093, -179.547) (115.1821, -179.4951) (115.0512, -179.4951) knots 0 0 0 1 2 2 2
  spline S187 degree 2 poles (115.0512, -179.4951) (114.7548, -179.4951) (114.4189, -179.9397) (114.4189, -180.3597) knots 0 0 0 1 2 2 2
  spline S188 degree 2 poles (114.4189, -180.3597) (114.4189, -180.7647) (114.6757, -181.192) (114.9598, -181.192) knots 0 0 0 1 2 2 2
  spline S189 degree 2 poles (114.9598, -181.192) (115.1105, -181.192) (115.4167, -181.0537) (115.5526, -180.9376) knots 0 0 0 1 2 2 2
  line L189 (118.2746, -181.4934) -> (117.8892, -181.4934)
  line L190 (117.8892, -181.4934) -> (117.8892, -181.2414)
  spline S190 degree 2 poles (117.8892, -181.2414) (117.7114, -181.3971) (117.3928, -181.5576) (117.1952, -181.5576) knots 0 0 0 1 2 2 2
  spline S191 degree 2 poles (117.1952, -181.5576) (117.047, -181.5576) (116.7827, -181.4588) (116.6863, -181.3526) knots 0 0 0 1 2 2 2
  spline S192 degree 2 poles (116.6863, -181.3526) (116.5875, -181.2464) (116.4789, -180.9228) (116.4789, -180.6906) knots 0 0 0 1 2 2 2
  line L191 (116.4789, -180.6906) -> (116.4789, -179.2062)
  line L192 (116.4789, -179.2062) -> (116.8642, -179.2062)
  line L193 (116.8642, -179.2062) -> (116.8642, -180.5103)
  spline S193 degree 2 poles (116.8642, -180.5103) (116.8642, -180.6931) (116.8913, -180.9327) (116.9383, -181.0216) knots 0 0 0 1 2 2 2
  spline S194 degree 2 poles (116.9383, -181.0216) (116.9852, -181.1105) (117.1458, -181.192) (117.2964, -181.192) knots 0 0 0 1 2 2 2
  spline S195 degree 2 poles (117.2964, -181.192) (117.4372, -181.192) (117.7559, -181.0315) (117.8892, -180.9154) knots 0 0 0 1 2 2 2
  line L194 (117.8892, -180.9154) -> (117.8892, -179.2062)
  line L195 (117.8892, -179.2062) -> (118.2746, -179.2062)
  line L196 (118.2746, -179.2062) -> (118.2746, -181.4934)
  spline S196 degree 2 poles (119.4503, -181.5477) (119.2206, -181.5477) (118.8229, -181.4242) (118.692, -181.3551) knots 0 0 0 1 2 2 2
  line L197 (118.692, -181.3551) -> (118.692, -180.9228)
  line L198 (118.692, -180.9228) -> (118.7117, -180.9228)
  spline S197 degree 2 poles (118.7117, -180.9228) (118.7611, -180.9623) (118.8945, -181.0562) (119.0057, -181.1081) knots 0 0 0 1 2 2 2
  spline S198 degree 2 poles (119.0057, -181.1081) (119.102, -181.155) (119.3391, -181.2242) (119.4651, -181.2242) knots 0 0 0 1 2 2 2
  spline S199 degree 2 poles (119.4651, -181.2242) (119.5565, -181.2242) (119.7664, -181.1822) (119.8158, -181.1476) knots 0 0 0 1 2 2 2
  spline S200 degree 2 poles (119.8158, -181.1476) (119.8875, -181.1007) (119.9517, -180.9944) (119.9517, -180.8858) knots 0 0 0 1 2 2 2
  spline S201 degree 2 poles (119.9517, -180.8858) (119.9517, -180.7499) (119.8035, -180.6091) (119.6133, -180.5622) knots 0 0 0 1 2 2 2
  spline S202 degree 2 poles (119.6133, -180.5622) (119.5392, -180.5449) (119.3021, -180.4955) (119.2008, -180.4683) knots 0 0 0 1 2 2 2
  spline S203 degree 2 poles (119.2008, -180.4683) (118.939, -180.3918) (118.7019, -180.0756) (118.7019, -179.8508) knots 0 0 0 1 2 2 2
  spline S204 degree 2 poles (118.7019, -179.8508) (118.7019, -179.5396) (119.1687, -179.1518) (119.554, -179.1518) knots 0 0 0 1 2 2 2
  spline S205 degree 2 poles (119.554, -179.1518) (119.7442, -179.1518) (120.1295, -179.2457) (120.2604, -179.3173) knots 0 0 0 1 2 2 2
  line L199 (120.2604, -179.3173) -> (120.2604, -179.7298)
  line L200 (120.2604, -179.7298) -> (120.2407, -179.7298)
  spline S206 degree 2 poles (120.2407, -179.7298) (120.0925, -179.6112) (119.7319, -179.4754) (119.5466, -179.4754) knots 0 0 0 1 2 2 2
  spline S207 degree 2 poles (119.5466, -179.4754) (119.3564, -179.4754) (119.0946, -179.6359) (119.0946, -179.7965) knots 0 0 0 1 2 2 2
  spline S208 degree 2 poles (119.0946, -179.7965) (119.0946, -179.9422) (119.2502, -180.083) (119.4231, -180.1275) knots 0 0 0 1 2 2 2
  spline S209 degree 2 poles (119.4231, -180.1275) (119.5071, -180.1497) (119.7195, -180.1942) (119.8356, -180.2213) knots 0 0 0 1 2 2 2
  spline S210 degree 2 poles (119.8356, -180.2213) (120.0875, -180.2856) (120.3444, -180.5795) (120.3444, -180.8339) knots 0 0 0 1 2 2 2
  spline S211 degree 2 poles (120.3444, -180.8339) (120.3444, -180.9821) (120.2283, -181.2439) (120.1147, -181.3402) knots 0 0 0 1 2 2 2
  spline S212 degree 2 poles (120.1147, -181.3402) (119.9937, -181.4415) (119.6849, -181.5477) (119.4503, -181.5477) knots 0 0 0 1 2 2 2
  spline S213 degree 2 poles (121.3942, -181.5378) (121.0805, -181.5378) (120.7273, -181.1797) (120.7273, -180.7919) knots 0 0 0 1 2 2 2
  line L201 (120.7273, -180.7919) -> (120.7273, -179.5248)
  line L202 (120.7273, -179.5248) -> (120.4679, -179.5248)
  line L203 (120.4679, -179.5248) -> (120.4679, -179.2062)
  line L204 (120.4679, -179.2062) -> (120.7273, -179.2062)
  line L205 (120.7273, -179.2062) -> (120.7273, -178.5491)
  line L206 (120.7273, -178.5491) -> (121.1126, -178.5491)
  line L207 (121.1126, -178.5491) -> (121.1126, -179.2062)
  line L208 (121.1126, -179.2062) -> (121.8215, -179.2062)
  line L209 (121.8215, -179.2062) -> (121.8215, -179.5248)
  line L210 (121.8215, -179.5248) -> (121.1126, -179.5248)
  line L211 (121.1126, -179.5248) -> (121.1126, -180.6141)
  spline S214 degree 2 poles (121.1126, -180.6141) (121.1126, -180.787) (121.125, -180.9772) (121.1669, -181.0587) knots 0 0 0 1 2 2 2
  spline S215 degree 2 poles (121.1669, -181.0587) (121.2015, -181.1303) (121.3571, -181.2019) (121.4905, -181.2019) knots 0 0 0 1 2 2 2
  spline S216 degree 2 poles (121.4905, -181.2019) (121.5844, -181.2019) (121.7597, -181.1451) (121.7993, -181.1278) knots 0 0 0 1 2 2 2
  line L212 (121.7993, -181.1278) -> (121.8215, -181.1278)
  line L213 (121.8215, -181.1278) -> (121.8215, -181.4736)
  spline S217 degree 2 poles (121.8215, -181.4736) (121.7128, -181.5033) (121.4905, -181.5378) (121.3942, -181.5378) knots 0 0 0 1 2 2 2
  line L214 (123.3183, -179.6186) -> (123.2986, -179.6186)
  spline S218 degree 2 poles (123.2986, -179.6186) (123.2541, -179.6063) (123.1578, -179.6014) (123.0911, -179.6014) knots 0 0 0 1 2 2 2
  spline S219 degree 2 poles (123.0911, -179.6014) (122.9355, -179.6014) (122.6292, -179.7372) (122.4909, -179.8706) knots 0 0 0 1 2 2 2
  line L215 (122.4909, -179.8706) -> (122.4909, -181.4934)
  line L216 (122.4909, -181.4934) -> (122.1055, -181.4934)
  line L217 (122.1055, -181.4934) -> (122.1055, -179.2062)
  line L218 (122.1055, -179.2062) -> (122.4909, -179.2062)
  line L219 (122.4909, -179.2062) -> (122.4909, -179.547)
  spline S220 degree 2 poles (122.4909, -179.547) (122.7008, -179.3593) (123.0145, -179.2062) (123.1627, -179.2062) knots 0 0 0 1 2 2 2
  spline S221 degree 2 poles (123.1627, -179.2062) (123.222, -179.2062) (123.2813, -179.2111) (123.3183, -179.2185) knots 0 0 0 1 2 2 2
  line L220 (123.3183, -179.2185) -> (123.3183, -179.6186)
  line L221 (124.0099, -181.4934) -> (123.6246, -181.4934)
  line L222 (123.6246, -181.4934) -> (123.6246, -179.2062)
  line L223 (123.6246, -179.2062) -> (124.0099, -179.2062)
  line L224 (124.0099, -179.2062) -> (124.0099, -181.4934)
  line L225 (124.0371, -178.8258) -> (123.5999, -178.8258)
  line L226 (123.5999, -178.8258) -> (123.5999, -178.4256)
  line L227 (123.5999, -178.4256) -> (124.0371, -178.4256)
  line L228 (124.0371, -178.4256) -> (124.0371, -178.8258)
  spline S222 degree 2 poles (125.5685, -181.5453) (125.0202, -181.5453) (124.4175, -180.9302) (124.4175, -180.3621) knots 0 0 0 1 2 2 2
  spline S223 degree 2 poles (124.4175, -180.3621) (124.4175, -179.8039) (125.0029, -179.1419) (125.4747, -179.1419) knots 0 0 0 1 2 2 2
  spline S224 degree 2 poles (125.4747, -179.1419) (125.6871, -179.1419) (126.0156, -179.2654) (126.1366, -179.3963) knots 0 0 0 1 2 2 2
  spline S225 degree 2 poles (126.1366, -179.3963) (126.2601, -179.5273) (126.391, -179.9052) (126.391, -180.1793) knots 0 0 0 1 2 2 2
  line L229 (126.391, -180.1793) -> (126.391, -180.3893)
  line L230 (126.391, -180.3893) -> (124.8077, -180.3893)
  spline S226 degree 2 poles (124.8077, -180.3893) (124.8077, -180.787) (125.2079, -181.2093) (125.5636, -181.2093) knots 0 0 0 1 2 2 2
  spline S227 degree 2 poles (125.5636, -181.2093) (125.6895, -181.2093) (125.9341, -181.1525) (126.0329, -181.1081) knots 0 0 0 1 2 2 2
  spline S228 degree 2 poles (126.0329, -181.1081) (126.1366, -181.0587) (126.2799, -180.9722) (126.3268, -180.9327) knots 0 0 0 1 2 2 2
  line L231 (126.3268, -180.9327) -> (126.349, -180.9327)